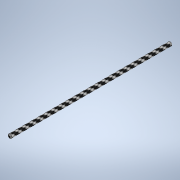
# Autodesk Inventor part: FlipperRod
Saved by Autodesk Inventor 2020 (Build 240168000, 168)
## iProperties
Created: 2023-12-22
Part Number: FlipperRod
Material: CFRP
Document SubType Name: Modeling
Designer: smz3rm
Density: 1.43 g/cm^3
Appearance: Carbon Fiber
Mass: 0.373198 g
Surface Area: 5.28239 cm^2
Volume: 0.260978 cm^3
Author: smz3rm
Autodesk Inventor part; units mm, degrees
ref_plane "YZ Plane" through (0, 0, 0) normal (1, 0, 0) x (0, 1, 0)
ref_plane "XZ Plane" through (0, 0, 0) normal (0, 1, 0) x (-1, 0, 0)
ref_plane "XY Plane" through (0, 0, 0) normal (0, 0, 1) x (1, 0, 0)
sketch "Sketch1" plane through (0, 0, 0) normal (0, 0, 1) x (1, 0, 0)
  circle A0 centre (0, 0) radius 1
  dimension "d0" = 2
  constraints: 1 centre point, 1 coincident
  measures "d0" diameter of A0
extrude "Extrusion1" add sketch "Sketch1" along normal blind 83.0718
equation "\"d0\" = FlipperRodDia"
equation "\"d1\" = FlipperRodLength"
equation "\"FlipperRodDia\" = 2"
equation "\"FlipperRodLength\" = 83.071797"
body "Solid1"
